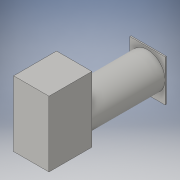
# Autodesk Inventor part: compressor
Saved by Autodesk Inventor 2016 (Build 200138000, 138)
## iProperties
Created: 2018-07-07
Part Number: compressor
Material: Generic
Document SubType Name: Modeling
Designer: Kade
Density: 1 g/cm^3
Appearance: Default
Author: Kade
Autodesk Inventor part; units mm, degrees
ref_plane "YZ Plane" through (0, 0, 0) normal (1, 0, 0) x (0, 1, 0)
ref_plane "XZ Plane" through (0, 0, 0) normal (0, 1, 0) x (-1, 0, 0)
ref_plane "XY Plane" through (0, 0, 0) normal (0, 0, 1) x (1, 0, 0)
sketch "Sketch1" plane through (0, 0, 0) normal (0, 1, 0) x (-1, 0, 0)
  line L0 (0, 0) -> (-88.9, 0)
  line L1 (-88.9, 0) -> (-88.9, -292.1)
  line L2 (-88.9, -292.1) -> (0, -292.1)
  line L3 (0, -292.1) -> (0, 0)
  dimension "d2" = 88.9
  dimension "d3" = 292.1
  constraints: 8 end point, 2 parallel, 1 horizontal, 1 perpendicular
  measures "d2" distance of L2.end L1.end
  measures "d3" distance of L1.end L0.end
extrude "Extrusion1" add sketch "Sketch1" along normal blind 165.1
sketch "Sketch2" plane through (88.9, 0, -292.1) normal (0, 0, -1) x (-1, 0, 0)
  line L0 (88.9, 165.1) -> (0, 165.1) projected
  line L1 (0, 0) -> (88.9, 0)
  line L2 (88.9, 0) -> (88.9, 165.1)
  line L3 (88.9, 165.1) -> (0, 165.1)
  line L4 (0, 165.1) -> (0, 0)
  circle A0 centre (44.45, 53.975) radius 44.45
  dimension "d6" = 44.45
  dimension "d7" = 88.9
  dimension "d8" = 53.975
  constraints: 8 end point, 2 parallel, 1 centre point, 1 horizontal, 1 perpendicular
  measures "d6" distance from line of L4 A0.centre
  measures "d7" diameter of A0
  measures "d8" distance from line of L1 A0.centre
extrude "Extrusion2" cut sketch "Sketch2" against normal blind 184.15 contours L2 A0 L4 L0 | L2 L1 L4 A0
sketch "Sketch3" plane through (44.45, 53.975, -292.1) normal (0, 0, -1) x (-1, 0, 0)
  line L0 (-44.3996, -53.975) -> (44.5004, -53.975)
  line L1 (44.5004, -53.975) -> (44.5004, 50.8)
  line L2 (44.5004, 50.8) -> (-44.3996, 50.8)
  line L3 (-44.3996, 50.8) -> (-44.3996, -53.975)
  point P0 (44.45, -53.975)
  dimension "d11" = 88.9
  dimension "d12" = 104.775
  constraints: 8 end point, 2 parallel, 1 horizontal, 1 perpendicular
  measures "d11" distance of L2.end L1.end
  measures "d12" distance of L1.end L0.end
extrude "Extrusion3" add sketch "Sketch3" along normal blind 3.175
body "Solid1"
